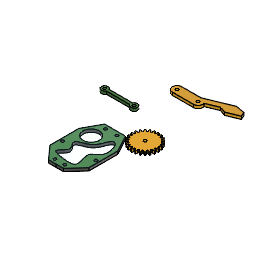
Robbotic gripper_ (Autodesk Fusion 360 design; units mm, degrees)
description: Spur Gear; Module: 1.125; Num Teeth: 24; Pressure Angle: 20.0; Backlash: 0.00 mm
Autodesk Fusion 360 part; units mm, degrees
note: some values were not read from the file. Set by a fixed rule: which sketch regions a step uses.
sketch "Sketch1" plane through (0, 0, 0) normal (0, 1, 0) x (1, 0, 0)
  line L0 (0, -5) -> (22, -5)
  arc A0 (22, -5) -> (22, 5) centre (22, 0) ccw
  line L1 (22, 5) -> (0, 5)
  arc A1 (0, 5) -> (0, -5) centre (0, 0) ccw
  line L2 (0, 0) -> (22, 0) construction
  line L3 (20.05, 5) -> (54.05, 18.9444)
  line L4 (54.05, 18.9444) -> (57.9834, 9.3537)
  line L5 (57.9834, 9.3537) -> (23.8973, -4.626)
  line L6 (46.4509, 15.8278) -> (56.0167, 14.1491)
  line L7 (26.7717, 1.4935) -> (39.0852, 6.5436)
  line L8 (39.0852, 6.5436) -> (45.4594, 4.2172)
  circle A2 centre (22, 0) radius 1.5
  circle A3 centre (0, 0) radius 1.5
  dimension "d1" = 22
  dimension "d2" = 10
  dimension "d3" = 157.7
  dimension "d4" = 34
  dimension "d5" = 1.95
  dimension "d6" = 3
  dimension "d7" = 3
  constraint tangent L0 A0
  constraint tangent A0 L1
  constraint parallel L0 L1
  constraint tangent L1 A1
  constraint tangent L0 A1
  constraint horizontal L2
  constraint coincident A1.centre L2.start
  constraint coincident L1 L3.start
  constraint perpendicular L3 L4
  constraint coincident A0 L5.end
  constraint tangent A0 L5
  constraint perpendicular L4 L5
  constraint coincident L3 L6.start
  constraint midpoint L4 L6.end
  constraint coincident A0 L7.start
  constraint coincident L5 L8.end
  constraint parallel L5 L7
  constraint concentric A0 A2
  constraint concentric A1 A3
  measures "d1" distance of A1.centre A0.centre
  measures "d2" diameter of A0
  measures "d3" angle of L1 L3
  measures "d4" horizontal distance of L3.start L3.end
  measures "d5" horizontal distance of A0.centre L3.start
  measures "d6" diameter of A2
  measures "d7" diameter of A3
extrude "Extrude1" add sketch "Sketch1" along normal blind 3 contours L0 A0 L1 A1 | A0 L1 L3 L4 L5 L6 L7 L8 makes body 1
sketch "Sketch2" plane through (0, 3, 0) normal (0, 1, 0) x (-1, 0, 0)
  circle A0 centre (0, 0) radius 1.5
  circle A1 centre (-22, 0) radius 1.5
  line L0 (-20.05, -5) -> (0, -5)
  arc A2 (0, -5) -> (0, 5) centre (0, 0) ccw
  line L1 (0, 5) -> (-22, 5)
  arc A3 (-22, 5) -> (-26.7717, -1.4935) centre (-22, 0) ccw
  line L2 (-26.7717, -1.4935) -> (-39.0852, -6.5436)
  line L3 (-39.0852, -6.5436) -> (-45.4594, -4.2172)
  line L4 (-45.4594, -4.2172) -> (-57.9834, -9.3537)
  line L5 (-57.9834, -9.3537) -> (-56.0167, -14.1491)
  line L6 (-56.0167, -14.1491) -> (-46.4509, -15.8278)
  line L7 (-46.4509, -15.8278) -> (-20.05, -5)
  circle A4 centre (14.9856, 15.0847) radius 3.5
  circle A5 centre (14.9856, 15.0847) radius 1.5
  line L8 (14.9856, 15.0847) -> (45.9856, 15.0847)
  circle A6 centre (45.9856, 15.0847) radius 1.5
  circle A7 centre (45.9856, 15.0847) radius 3.5
  line L9 (18.1479, 16.5847) -> (42.8233, 16.5847)
  line L10 (18.1479, 13.5847) -> (42.8233, 13.5847)
  dimension "d12" = 3
  dimension "d13" = 7
  dimension "d14" = 3
  dimension "d15" = 7
  dimension "d16" = 31
  dimension "d17" = 1.5
  constraint concentric A4 A5
  constraint coincident A4.centre A5.centre
  constraint horizontal L8
  constraint coincident L8.end A6.centre
  constraint coincident A4 L9.start
  constraint coincident A7 L9.end
  constraint horizontal L9
  constraint symmetric L8 L9.start L10.start
  constraint symmetric L8 L9.end L10.end
  measures "d12" diameter of A5
  measures "d13" diameter of A4
  measures "d14" diameter of A6
  measures "d15" diameter of A7
  measures "d16" distance of A4.centre L8.end
  measures "d17" distance of L8 L9
extrude "Extrude2" add sketch "Sketch2" along normal blind 3 separate body contours A4 | A4 L8 A7 L10 | A4 L8 A7 L9 | A7 makes body 2
sketch "Sketch3" plane through (0, 6, 0) normal (0, 1, 0) x (-1, 0, 0)
  circle A0 centre (45.9856, 15.0847) radius 1.5
  line L0 (18.1479, 13.5847) -> (42.8233, 13.5847)
  arc A1 (42.8233, 13.5847) -> (42.8233, 16.5847) centre (45.9856, 15.0847) ccw
  line L1 (42.8233, 16.5847) -> (18.1479, 16.5847)
  line L2 (-0.3311, 50.4983) -> (-0.3311, 112.4983)
  line L3 (-0.3311, 50.4983) -> (-11.3311, 50.4983)
  line L4 (-11.3311, 50.4983) -> (-20.8311, 68.098)
  line L5 (-20.8311, 68.098) -> (-20.8311, 98.398)
  line L6 (-20.8311, 98.398) -> (-8.2649, 112.4484)
  line L7 (-8.2649, 112.4484) -> (-0.3311, 112.4983)
  circle A2 centre (-6.3311, 54.4983) radius 1.5
  circle A3 centre (-17.8119, 88.098) radius 1.5
  circle A4 centre (-5.5149, 108.4656) radius 1.5
  circle A5 centre (17.1498, 88.098) radius 1.5
  line L8 (10.6689, 50.4983) -> (20.1689, 68.098)
  line L9 (-0.3311, 50.4983) -> (-0.3311, 112.4983)
  line L10 (-0.3311, 50.4983) -> (10.6689, 50.4983)
  line L11 (7.6027, 112.4484) -> (-0.3311, 112.4983)
  line L12 (20.1689, 68.098) -> (20.1689, 98.398)
  circle A6 centre (5.6689, 54.4983) radius 1.5
  line L13 (20.1689, 98.398) -> (7.6027, 112.4484)
  circle A7 centre (4.8527, 108.4656) radius 1.5
  circle A8 centre (7.1689, 68.098) radius 8.5
  line L14 (20.1689, 68.098) -> (-0.3311, 68.098)
  dimension "d54" = 62
  dimension "d55" = 11
  dimension "d56" = 20
  dimension "d57" = 30.3
  dimension "d58" = 18.85
  dimension "d59" = 20.5
  dimension "d60" = 3
  dimension "d61" = 3
  dimension "d62" = 3
  dimension "d63" = 6
  dimension "d64" = 4
  dimension "d65" = 10.3
  dimension "d66" = 4
  dimension "d67" = 2.75
  dimension "d68" = 17
  dimension "d69" = 13
  constraint vertical L2
  constraint perpendicular L2 L3
  constraint perpendicular L3 L5
  constraint symmetric L3.start L2 L9.start
  constraint symmetric L7.end L2 L9.end
  constraint symmetric L2 L3.end L8.start
  constraint symmetric L2 L4.end L8.end
  constraint symmetric L2 L5.end L12.end
  constraint symmetric L2 L6.end L11.start
  constraint symmetric L2 A2 A6
  constraint symmetric L2 A3 A5
  constraint symmetric L2 A4 A7
  constraint coincident L9 L14.end
  constraint perpendicular L9 L14
  constraint coincident A8.centre L14
  measures "d54" distance of L2.start L2.end
  measures "d55" distance of L2.start L3.end
  measures "d56" distance of L3.end L4.end
  measures "d57" distance of L4.end L5.end
  measures "d58" distance of L5.end L6.end
  measures "d59" distance of L2 L5
  measures "d60" diameter of A2
  measures "d61" diameter of A3
  measures "d62" diameter of A4
  measures "d63" distance of L2 A2.centre
  measures "d64" distance of L3 A2.centre
  measures "d65" vertical distance of L5.end A3.centre
  measures "d66" distance of L7 A4.centre
  measures "d67" horizontal distance of L6.end A4.centre
  measures "d68" diameter of A8
  measures "d69" distance of L8.end A8.centre
extrude "Extrude3" add sketch "Sketch3" along normal blind 3 separate body contours L2 L3 L4 L5 L6 L7 L9 A8 | L2 L8 L9 L10 A8 L14 | L2 L9 L11 L12 L13 A8 L14 makes body 3
sketch "Sketch4" plane through (0, 9, 0) normal (0, 1, 0) x (-1, 0, 0)
  circle A0 centre (5.6689, 54.4983) radius 1.5
  circle A1 centre (-6.3311, 54.4983) radius 1.5
  circle A2 centre (-5.5149, 108.4656) radius 1.5
  circle A3 centre (17.1498, 88.098) radius 1.5
  circle A4 centre (-17.8119, 88.098) radius 1.5
  circle A5 centre (7.1689, 68.098) radius 8.5
  circle A6 centre (4.8527, 108.4656) radius 1.5
  line L0 (-11.3311, 50.4983) -> (10.6689, 50.4983)
  line L1 (10.6689, 50.4983) -> (20.1689, 68.098)
  line L2 (20.1689, 68.098) -> (20.1689, 98.398)
  line L3 (20.1689, 98.398) -> (7.6027, 112.4484)
  line L4 (7.6027, 112.4484) -> (-0.3311, 112.4983)
  line L5 (-0.3311, 112.4983) -> (-8.2649, 112.4484)
  line L6 (-8.2649, 112.4484) -> (-20.8311, 98.398)
  line L7 (-20.8311, 98.398) -> (-20.8311, 68.098)
  line L8 (-20.8311, 68.098) -> (-11.3311, 50.4983)
  spline S0 degree 5 poles (-16.085, 78.7784) (-16.298, 78.2987) (-16.6612, 77.27) (-17.0001, 75.5207) (-17.0066, 72.8404) (-16.3269, 69.2714) (-15.1093, 65.9488) (-13.5574, 63.3457) (-11.8859, 61.8449) (-10.2795, 61.6482) (-8.8477, 62.6646) (-7.6253, 64.5932) (-6.5802, 67.0369) (-5.6199, 69.5977) (-4.5923, 71.998) (-3.3223, 74.0928) (-1.662, 75.8343) (0.4595, 77.2515) (2.9926, 78.4238) (5.7048, 79.457) (8.178, 80.4608) (9.9631, 81.5391) (10.7157, 82.776) (10.3197, 84.2251) (9.0651, 85.894) (7.5463, 87.7491) (6.4185, 89.7295) (6.2135, 91.7586) (7.1002, 93.7562) (8.7579, 95.6492) (10.6021, 97.3763) (11.9622, 98.894) (12.2609, 100.1807) (11.2342, 101.2453) (8.9526, 102.1186) (5.7032, 102.8331) (1.9147, 103.4073) (-1.9363, 103.8263) (-5.4087, 104.0262) (-8.1899, 103.8729) (-10.0993, 103.208) (-11.0856, 101.904) (-11.2236, 99.9108) (-10.718, 97.3193) (-9.8838, 94.3741) (-9.0758, 91.3848) (-8.6301, 88.6603) (-8.7982, 86.4293) (-9.6913, 84.7776) (-11.1999, 83.5504) (-13.0372, 82.4147) (-14.479, 81.2755) (-15.3832, 80.1486) (-15.872, 79.2582) (-16.085, 78.7784) knots 0 0 0 0 0 0 0.02 0.04 0.06 0.08 0.1 0.12 0.14 0.16 0.18 0.2 0.22 0.24 0.26 0.28 0.3 0.32 0.34 0.36 0.38 0.4 0.42 0.44 0.46 0.48 0.5 0.52 0.54 0.56 0.58 0.6 0.62 0.64 0.66 0.68 0.7 0.72 0.74 0.76 0.78 0.8 0.82 0.84 0.86 0.88 0.9 0.92 0.94 0.96 0.98 1 1 1 1 1 1
  point P0 (-11.6817, 62.0657)
  point P1 (-6.2775, 67.8701)
  point P2 (2.3291, 78.0779)
  point P3 (10.4353, 83.2819)
  point P4 (6.4322, 91.288)
  point P5 (11.9364, 99.3942)
  point P6 (-2.1744, 103.7976)
  point P7 (-11.0812, 100.495)
  point P8 (-9.1797, 85.9839)
extrude "Extrude4" cut sketch "Sketch4" against normal blind 10 contours S0 bodies 3
sketch "Base Circle" plane through (0, 0, 0) normal (0, 0, 1) x (1, 0, 0)
  circle A0 centre (0, 0) radius 12.1984
  circle A1 centre (0, 0) radius 1.5
sketch "Gear Tooth" plane through (0, 0, 0) normal (0, 0, 1) x (1, 0, 0)
sketch "Diametrial Pitch Circle" plane through (0, 0, 0) normal (0, 0, 1) x (1, 0, 0)
sketch "Sketch8" plane through (0, 9, 0) normal (0, 1, 0) x (-1, 0, 0)
  spline S0 degree 5 poles (-16.085, 78.7784) (-15.872, 79.2582) (-15.3832, 80.1486) (-14.479, 81.2755) (-13.0372, 82.4147) (-11.1999, 83.5504) (-9.6913, 84.7776) (-8.7982, 86.4293) (-8.6301, 88.6603) (-9.0758, 91.3848) (-9.8838, 94.3741) (-10.718, 97.3193) (-11.2236, 99.9108) (-11.0856, 101.904) (-10.0993, 103.208) (-8.1899, 103.8729) (-5.4087, 104.0262) (-1.9363, 103.8263) (1.9147, 103.4073) (5.7032, 102.8331) (8.9526, 102.1186) (11.2342, 101.2453) (12.2609, 100.1807) (11.9622, 98.894) (10.6021, 97.3763) (8.7579, 95.6492) (7.1002, 93.7562) (6.2135, 91.7586) (6.4185, 89.7295) (7.5463, 87.7491) (9.0651, 85.894) (10.3197, 84.2251) (10.7157, 82.776) (9.9631, 81.5391) (8.178, 80.4608) (5.7048, 79.457) (2.9926, 78.4238) (0.4595, 77.2515) (-1.662, 75.8343) (-3.3223, 74.0928) (-4.5923, 71.998) (-5.6199, 69.5977) (-6.5802, 67.0369) (-7.6253, 64.5932) (-8.8477, 62.6646) (-10.2795, 61.6482) (-11.8859, 61.8449) (-13.5574, 63.3457) (-15.1093, 65.9488) (-16.3269, 69.2714) (-17.0066, 72.8404) (-17.0001, 75.5207) (-16.6612, 77.27) (-16.298, 78.2987) (-16.085, 78.7784) knots -1 -1 -1 -1 -1 -1 -0.98 -0.96 -0.94 -0.92 -0.9 -0.88 -0.86 -0.84 -0.82 -0.8 -0.78 -0.76 -0.74 -0.72 -0.7 -0.68 -0.66 -0.64 -0.62 -0.6 -0.58 -0.56 -0.54 -0.52 -0.5 -0.48 -0.46 -0.44 -0.42 -0.4 -0.38 -0.36 -0.34 -0.32 -0.3 -0.28 -0.26 -0.24 -0.22 -0.2 -0.18 -0.16 -0.14 -0.12 -0.1 -0.08 -0.06 -0.04 -0.02 0 0 0 0 0 0
  circle A0 centre (5.6689, 54.4983) radius 1.5
  circle A1 centre (-6.3311, 54.4983) radius 1.5
  circle A2 centre (-5.5149, 108.4656) radius 1.5
  circle A3 centre (17.1498, 88.098) radius 1.5
  circle A4 centre (-17.8119, 88.098) radius 1.5
  circle A5 centre (7.1689, 68.098) radius 8.5
  circle A6 centre (4.8527, 108.4656) radius 1.5
  line L0 (-11.3311, 50.4983) -> (10.6689, 50.4983)
  line L1 (10.6689, 50.4983) -> (20.1689, 68.098)
  line L2 (20.1689, 68.098) -> (20.1689, 98.398)
  line L3 (20.1689, 98.398) -> (7.6027, 112.4484)
  line L4 (7.6027, 112.4484) -> (-0.3311, 112.4983)
  line L5 (-0.3311, 112.4983) -> (-8.2649, 112.4484)
  line L6 (-8.2649, 112.4484) -> (-20.8311, 98.398)
  line L7 (-20.8311, 98.398) -> (-20.8311, 68.098)
  line L8 (-20.8311, 68.098) -> (-11.3311, 50.4983)
sketch "Sketch9" plane through (0, 0, 0) normal (0, 1, 0) x (1, 0, 0)
sketch "Sketch10" plane through (0, 9, 0) normal (0, 1, 0) x (-1, 0, 0)
  spline S0 degree 5 poles (-16.085, 78.7784) (-15.872, 79.2582) (-15.3832, 80.1486) (-14.479, 81.2755) (-13.0372, 82.4147) (-11.1999, 83.5504) (-9.6913, 84.7776) (-8.7982, 86.4293) (-8.6301, 88.6603) (-9.0758, 91.3848) (-9.8838, 94.3741) (-10.718, 97.3193) (-11.2236, 99.9108) (-11.0856, 101.904) (-10.0993, 103.208) (-8.1899, 103.8729) (-5.4087, 104.0262) (-1.9363, 103.8263) (1.9147, 103.4073) (5.7032, 102.8331) (8.9526, 102.1186) (11.2342, 101.2453) (12.2609, 100.1807) (11.9622, 98.894) (10.6021, 97.3763) (8.7579, 95.6492) (7.1002, 93.7562) (6.2135, 91.7586) (6.4185, 89.7295) (7.5463, 87.7491) (9.0651, 85.894) (10.3197, 84.2251) (10.7157, 82.776) (9.9631, 81.5391) (8.178, 80.4608) (5.7048, 79.457) (2.9926, 78.4238) (0.4595, 77.2515) (-1.662, 75.8343) (-3.3223, 74.0928) (-4.5923, 71.998) (-5.6199, 69.5977) (-6.5802, 67.0369) (-7.6253, 64.5932) (-8.8477, 62.6646) (-10.2795, 61.6482) (-11.8859, 61.8449) (-13.5574, 63.3457) (-15.1093, 65.9488) (-16.3269, 69.2714) (-17.0066, 72.8404) (-17.0001, 75.5207) (-16.6612, 77.27) (-16.298, 78.2987) (-16.085, 78.7784) knots -1 -1 -1 -1 -1 -1 -0.98 -0.96 -0.94 -0.92 -0.9 -0.88 -0.86 -0.84 -0.82 -0.8 -0.78 -0.76 -0.74 -0.72 -0.7 -0.68 -0.66 -0.64 -0.62 -0.6 -0.58 -0.56 -0.54 -0.52 -0.5 -0.48 -0.46 -0.44 -0.42 -0.4 -0.38 -0.36 -0.34 -0.32 -0.3 -0.28 -0.26 -0.24 -0.22 -0.2 -0.18 -0.16 -0.14 -0.12 -0.1 -0.08 -0.06 -0.04 -0.02 0 0 0 0 0 0
  circle A0 centre (5.6689, 54.4983) radius 1.5
  circle A1 centre (-6.3311, 54.4983) radius 1.5
  circle A2 centre (-5.5149, 108.4656) radius 1.5
  circle A3 centre (17.1498, 88.098) radius 1.5
  circle A4 centre (-17.8119, 88.098) radius 1.5
  circle A5 centre (7.1689, 68.098) radius 8.5
  circle A6 centre (4.8527, 108.4656) radius 1.5
  line L0 (-11.3311, 50.4983) -> (10.6689, 50.4983)
  line L1 (10.6689, 50.4983) -> (20.1689, 68.098)
  line L2 (20.1689, 68.098) -> (20.1689, 98.398)
  line L3 (20.1689, 98.398) -> (7.6027, 112.4484)
  line L4 (7.6027, 112.4484) -> (-0.3311, 112.4983)
  line L5 (-0.3311, 112.4983) -> (-8.2649, 112.4484)
  line L6 (-8.2649, 112.4484) -> (-20.8311, 98.398)
  line L7 (-20.8311, 98.398) -> (-20.8311, 68.098)
  line L8 (-20.8311, 68.098) -> (-11.3311, 50.4983)
sketch "Base Circle (1)" plane through (0, 0, 0) normal (0, 0, 1) x (1, 0, 0)
  circle A0 centre (0, 0) radius 12.1984
  circle A1 centre (0, 0) radius 1.5
extrude "Extrude7" add sketch "Base Circle (1)" along normal blind 3 separate body makes body 4
sketch "Gear Tooth (1)" plane through (0, 0, 0) normal (0, 0, 1) x (1, 0, 0)
  spline S0 degree 5 poles (12.6449, -1.0183) (12.6506, -1.0187) (12.6618, -1.0195) (12.6788, -1.0202) (12.7014, -1.0204) (12.7297, -1.0195) (12.758, -1.0178) (12.7864, -1.0156) (12.8147, -1.0131) (12.8431, -1.0105) (12.8715, -1.0076) (12.8999, -1.0045) (12.9284, -1.0011) (12.9568, -0.9973) (12.9852, -0.9932) (13.0137, -0.9886) (13.0421, -0.9838) (13.0705, -0.9787) (13.099, -0.9733) (13.1274, -0.9678) (13.1559, -0.962) (13.1843, -0.956) (13.2127, -0.9498) (13.2412, -0.9433) (13.2696, -0.9366) (13.298, -0.9297) (13.3264, -0.9226) (13.3549, -0.9152) (13.3833, -0.9076) (13.4117, -0.8999) (13.4401, -0.8919) (13.4684, -0.8838) (13.4968, -0.8754) (13.5252, -0.8669) (13.5535, -0.8581) (13.5819, -0.8492) (13.6102, -0.8401) (13.6385, -0.8308) (13.6669, -0.8214) (13.6952, -0.8117) (13.7234, -0.8019) (13.7517, -0.7919) (13.78, -0.7817) (13.8082, -0.7714) (13.8365, -0.7609) (13.8647, -0.7502) (13.8929, -0.7393) (13.9211, -0.7283) (13.9492, -0.7171) (13.9774, -0.7058) (14.0055, -0.6943) (14.0337, -0.6826) (14.0618, -0.6708) (14.0898, -0.6588) (14.1179, -0.6467) (14.146, -0.6344) (14.174, -0.6219) (14.202, -0.6093) (14.23, -0.5966) (14.2579, -0.5837) (14.2859, -0.5706) (14.3138, -0.5574) (14.3417, -0.544) (14.3696, -0.5305) (14.3975, -0.5169) (14.4253, -0.5031) (14.4531, -0.4891) (14.4809, -0.4751) (14.5087, -0.4608) (14.5364, -0.4465) (14.5641, -0.4319) (14.5863, -0.4202) (14.6029, -0.4114) (14.6139, -0.4054) (14.6195, -0.4024) knots 0 0 0 0 0 0 0.01428571 0.02857143 0.04285714 0.05714286 0.07142857 0.08571429 0.1 0.11428571 0.12857143 0.14285714 0.15714286 0.17142857 0.18571429 0.2 0.21428571 0.22857143 0.24285714 0.25714286 0.27142857 0.28571429 0.3 0.31428571 0.32857143 0.34285714 0.35714286 0.37142857 0.38571429 0.4 0.41428571 0.42857143 0.44285714 0.45714286 0.47142857 0.48571429 0.5 0.51428571 0.52857143 0.54285714 0.55714286 0.57142857 0.58571429 0.6 0.61428571 0.62857143 0.64285714 0.65714286 0.67142857 0.68571429 0.7 0.71428571 0.72857143 0.74285714 0.75714286 0.77142857 0.78571429 0.8 0.81428571 0.82857143 0.84285714 0.85714286 0.87142857 0.88571429 0.9 0.91428571 0.92857143 0.94285714 0.95714286 0.97142857 0.98571429 1 1 1 1 1 1
  spline S1 degree 5 poles (12.6449, 1.0183) (12.6506, 1.0187) (12.6618, 1.0195) (12.6788, 1.0202) (12.7014, 1.0204) (12.7297, 1.0195) (12.758, 1.0178) (12.7864, 1.0156) (12.8147, 1.0131) (12.8431, 1.0105) (12.8715, 1.0076) (12.8999, 1.0045) (12.9284, 1.0011) (12.9568, 0.9973) (12.9852, 0.9932) (13.0137, 0.9886) (13.0421, 0.9838) (13.0705, 0.9787) (13.099, 0.9733) (13.1274, 0.9678) (13.1559, 0.962) (13.1843, 0.956) (13.2127, 0.9498) (13.2412, 0.9433) (13.2696, 0.9366) (13.298, 0.9297) (13.3264, 0.9226) (13.3549, 0.9152) (13.3833, 0.9076) (13.4117, 0.8999) (13.4401, 0.8919) (13.4684, 0.8838) (13.4968, 0.8754) (13.5252, 0.8669) (13.5535, 0.8581) (13.5819, 0.8492) (13.6102, 0.8401) (13.6385, 0.8308) (13.6669, 0.8214) (13.6952, 0.8117) (13.7234, 0.8019) (13.7517, 0.7919) (13.78, 0.7817) (13.8082, 0.7714) (13.8365, 0.7609) (13.8647, 0.7502) (13.8929, 0.7393) (13.9211, 0.7283) (13.9492, 0.7171) (13.9774, 0.7058) (14.0055, 0.6943) (14.0337, 0.6826) (14.0618, 0.6708) (14.0898, 0.6588) (14.1179, 0.6467) (14.146, 0.6344) (14.174, 0.6219) (14.202, 0.6093) (14.23, 0.5966) (14.2579, 0.5837) (14.2859, 0.5706) (14.3138, 0.5574) (14.3417, 0.544) (14.3696, 0.5305) (14.3975, 0.5169) (14.4253, 0.5031) (14.4531, 0.4891) (14.4809, 0.4751) (14.5087, 0.4608) (14.5364, 0.4465) (14.5641, 0.4319) (14.5863, 0.4202) (14.6029, 0.4114) (14.6139, 0.4054) (14.6195, 0.4024) knots 0 0 0 0 0 0 0.01428571 0.02857143 0.04285714 0.05714286 0.07142857 0.08571429 0.1 0.11428571 0.12857143 0.14285714 0.15714286 0.17142857 0.18571429 0.2 0.21428571 0.22857143 0.24285714 0.25714286 0.27142857 0.28571429 0.3 0.31428571 0.32857143 0.34285714 0.35714286 0.37142857 0.38571429 0.4 0.41428571 0.42857143 0.44285714 0.45714286 0.47142857 0.48571429 0.5 0.51428571 0.52857143 0.54285714 0.55714286 0.57142857 0.58571429 0.6 0.61428571 0.62857143 0.64285714 0.65714286 0.67142857 0.68571429 0.7 0.71428571 0.72857143 0.74285714 0.75714286 0.77142857 0.78571429 0.8 0.81428571 0.82857143 0.84285714 0.85714286 0.87142857 0.88571429 0.9 0.91428571 0.92857143 0.94285714 0.95714286 0.97142857 0.98571429 1 1 1 1 1 1
  arc A0 (14.6195, -0.4024) -> (14.6195, 0.4024) centre (0, 0) ccw
  line L0 (12.149, -0.9783) -> (12.6449, -1.0183)
  line L1 (12.149, 0.9783) -> (12.6449, 1.0183)
  line L2 (12.149, -0.9783) -> (12.149, 0.9783)
  point P0 (12.7841, -1.0157)
  point P1 (12.9241, -1.0016)
  point P2 (13.0647, -0.9797)
  point P3 (13.2057, -0.9513)
  point P4 (13.3469, -0.9172)
  point P5 (13.4884, -0.8779)
  point P6 (13.63, -0.8336)
  point P7 (13.7716, -0.7847)
  point P8 (13.9132, -0.7313)
  point P9 (14.0548, -0.6737)
  point P10 (14.1963, -0.6119)
  point P11 (14.3376, -0.546)
  point P12 (14.4787, -0.4761)
  point P13 (12.7841, 1.0157)
  point P14 (12.9241, 1.0016)
  point P15 (13.0647, 0.9797)
  point P16 (13.2057, 0.9513)
  point P17 (13.3469, 0.9172)
  point P18 (13.4884, 0.8779)
  point P19 (13.63, 0.8336)
  point P20 (13.7716, 0.7847)
  point P21 (13.9132, 0.7313)
  point P22 (14.0548, 0.6737)
  point P23 (14.1963, 0.6119)
  point P24 (14.3376, 0.546)
  point P25 (14.4787, 0.4761)
extrude "Extrude8" add sketch "Gear Tooth (1)" along normal blind 3 bodies 4
fillet "Fillet2" radius 0.1 2 edges at (12.159, -0.9791, 1.5) (12.159, 0.9791, 1.5) on bodies 4
pattern_circular "C-Pattern2" count 24 over 360 about axis through (0, 0, 0) along (0, 0, 1) of "Extrude8", "Fillet2"
sketch "Diametrial Pitch Circle (1)" plane through (0, 0, 0) normal (0, 0, 1) x (1, 0, 0)
move_body "Move1" bodies 4 to x (1, 0, 0) y (0, 0, 1) z (0, -1, 0) at (3, 15.7255, 20.2745)
sketch "Sketch14" plane through (0, 0, 0) normal (0, 1, 0) x (1, 0, 0)
move_body "Move2" bodies 1 to x (1, 0, 0) y (0, 1, 0) z (0, 0, 1) at (15, 0, 0)
move_body "Move3" bodies 1 to x (1, 0, 0) y (0, 1, 0) z (0, 0, 1) at (0, 25, 0)
move_body "Move4" bodies 4 to x (1, 0, 0) y (0, 1, 0) z (0, 0, 1) at (36.8624, 7.2951, 38.2639)
named bodies: "Spur Gear (24 teeth)"
